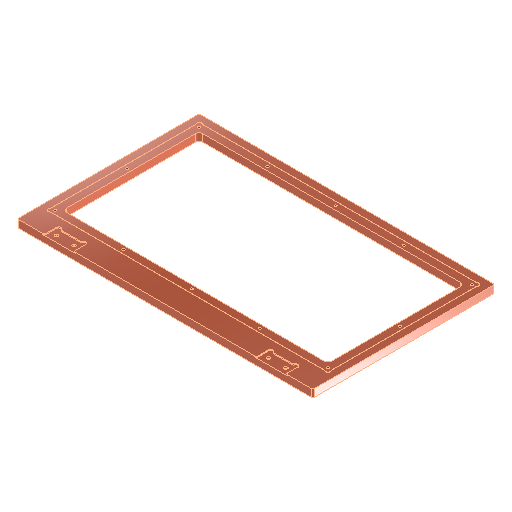
# Autodesk Inventor part: GRJ-04-105
Saved by Autodesk Inventor 2026.1 (Build 301233000, 233)
## iProperties
Company: Gree
Created: 2025-09-10
Part Number: GRJ-04-105
Material: Fenolite OR
Document SubType Name: Modeling
Designer: Willian Pinheiro
Density: 1.38 g/cm^3
Appearance: Suave - Laranja claro
Description: Suporte Estencil Principal
Project: GRJ-04
Mass: 415.457 g
Surface Area: 856.465 cm^2
Volume: 301.056 cm^3
Checked By: Antonio Lucas
Engr Approved By: Antonio Lucas
Mfg Approved By: Anderson Oliveira
Total: 1
Dimensões: 10 x 240 x 390 mm
Author: Willian Pinheiro
Title: Pasta Dissipador G
Revision Number: 00
Autodesk Inventor part; units mm, degrees
ref_plane "YZ Plane" through (0, 0, 0) normal (1, 0, 0) x (0, 1, 0)
ref_plane "XZ Plane" through (0, 0, 0) normal (0, 1, 0) x (-1, 0, 0)
ref_plane "XY Plane" through (0, 0, 0) normal (0, 0, 1) x (1, 0, 0)
sketch "Esboço1" plane through (0, 0, 0) normal (0, 0, 1) x (1, 0, 0)
  line L0 (-195, -120) -> (-195, 120)
  line L1 (-195, 120) -> (195, 120)
  line L2 (195, 120) -> (195, -120)
  line L3 (195, -120) -> (-195, -120)
  line L4 (0, 168.2) -> (0, -169.2) construction
  line L5 (-273, 0) -> (273, 0) construction
  line L6 (175, 100) -> (175, -80)
  line L7 (175, -80) -> (-175, -80)
  line L8 (-175, -80) -> (-175, 100)
  line L9 (-175, 100) -> (175, 100)
  line L10 (185, 110) -> (185, -90) construction
  line L11 (185, -90) -> (-185, -90) construction
  line L12 (-185, -90) -> (-185, 110) construction
  line L13 (-185, 110) -> (185, 110) construction
  line L14 (185.25, 110.25) -> (185.25, -90.25)
  line L15 (185.25, -90.25) -> (-185.25, -90.25)
  line L16 (-185.25, -90.25) -> (-185.25, 110.25)
  line L17 (-185.25, 110.25) -> (185.25, 110.25)
  circle A0 centre (183.25, 108.25) radius 3
  circle A1 centre (-183.25, 108.25) radius 3
  line L18 (175, 10) -> (-175, 10) construction
  circle A2 centre (183.25, -88.25) radius 3
  circle A3 centre (-183.25, -88.25) radius 3
  line L19 (180, 105) -> (180, -85) construction
  line L20 (180, -85) -> (-180, -85) construction
  line L21 (-180, -85) -> (-180, 105) construction
  line L22 (-180, 105) -> (180, 105) construction
  line L23 (159.5, -104) -> (159.5, -120)
  line L24 (159.5, -120) -> (120.5, -120)
  line L25 (120.5, -120) -> (120.5, -104)
  line L26 (120.5, -104) -> (159.5, -104)
  line L27 (140, -104) -> (140, -120) construction
  line L28 (159.5, -112) -> (120.5, -112) construction
  circle A4 centre (123.5, -104) radius 3
  line L29 (-159.5, -104) -> (-159.5, -120)
  line L30 (-159.5, -120) -> (-120.5, -120)
  line L31 (-120.5, -120) -> (-120.5, -104)
  line L32 (-120.5, -104) -> (-159.5, -104)
  line L33 (-140, -105) -> (-140, -121) construction
  line L34 (-159.5, -112) -> (-120.5, -112) construction
  circle A5 centre (-156.5, -104) radius 3
  circle A6 centre (-123.5, -104) radius 3
  circle A7 centre (156.5, -104) radius 3
  point P0 (0, 0)
  point P1 (0, -85)
  point P2 (-180, 10)
  point P3 (180, 10)
  point P4 (0, 105)
  point P5 (151.5, -112)
  point P6 (128.5, -112)
  point P7 (-151.5, -112)
  point P8 (-128.5, -112)
  point P9 (-181.0139, 110.25)
  point P10 (-185.25, 106.0139)
  point P11 (-185.25, -86.0139)
  point P12 (-181.0139, -90.25)
  point P13 (181.0139, -90.25)
  point P14 (185.25, -86.0139)
  point P15 (185.25, 106.0139)
  point P16 (181.0139, 110.25)
  point P17 (159.5, -120)
  point P18 (126.5, -104)
  point P19 (-153.5, -104)
  point P20 (-159.5, -120)
  point P21 (-126.5, -104)
  point P22 (-90, 105)
  point P23 (90, 105)
  point P24 (-90, -85)
  point P25 (90, -85)
  point P26 (106.5, -104)
  point P27 (153.5, -104)
  dimension "d112" = 10
  dimension "d113" = 0.25
  dimension "d114" = 6
  dimension "d115" = 2
  dimension "d116" = 2
  dimension "d117" = 5
  dimension "d123" = 16
  dimension "d124" = 8
  dimension "d125" = 39
  dimension "d126" = 280
  dimension "d127" = 240
  dimension "d128" = 390
  dimension "d129" = 20
  dimension "d130" = 200
  dimension "d131" = 350
  dimension "d132" = 10
  dimension "d133" = 0.25
  dimension "d134" = 5
  dimension "d163" = 90
  dimension "d164" = 90
  dimension "d165" = 23
  dimension "d166" = 370
  constraints: 62 end point, 12 midpoint, 7 centre point, 7 symmetric about line, 5 point on line, 4 coincident, 3 horizontal, 2 collinear, 1 parallel, 1 tangent, 28 other
  measures "d112" distance between parallel lines of L9 L13
  measures "d113" distance between parallel lines of L17 L13
  measures "d114" diameter of A0
  measures "d115" distance from line of A0.centre L17
  measures "d116" distance from line of A0.centre L14
  measures "d117" distance between parallel lines of L22 L9
  measures "d124" distance between parallel lines of L3 L34
  measures "d125" distance between parallel lines of L31 L29
  measures "d126" distance between parallel lines of L27 L33
  measures "d127" distance between parallel lines of L1 L3
  measures "d128" distance between parallel lines of L2 L0
  measures "d129" distance between parallel lines of L9 L1
  measures "d130" distance between parallel lines of L7 L1
  measures "d131" distance between parallel lines of L6 L8
  measures "d132" distance between parallel lines of L12 L8
  measures "d133" distance between parallel lines of L16 L12
  measures "d134" distance between parallel lines of L21 L8
  measures "d163" distance from line of point (-90, 105) L21
  measures "d164" distance of point (0, 105) point (-90, 105)
  measures "d165" distance of point (-128.5, -112) point (-151.5, -112)
  measures "d166" distance between parallel lines of L12 L10
extrude "Extrusão1" add sketch "Esboço1" against normal blind 10 contours L0 L1 L2 L3 L23 A7 L26 A4 L25 L31 A6 L32 A5 L29 | L29 A5 L32 A6 L31 L3 | A5 L32 | L32 A5 | L25 A4 L26 A7 L23 L3 | A6 L32 | L32 A6 | A4 L26 | L26 A4 | A7 L26 | L26 A7 | L6 L7 L8 L9 | L17 A0 L14 | L14 A0 L17 | L14 A2 L15 A3 L16 A1 L17 A0 | A2 L15 L14 | L14 L15 A2 | A1 L16 L17 | L17 L16 A1 | A3 L16 L15 | L15 L16 A3
extrude "Extrusion13" cut sketch "Esboço1" against normal blind 0.2 contours L6 L7 L8 L9 | L17 A0 L14 | L14 A0 L17 | L14 A2 L15 A3 L16 A1 L17 A0 | A2 L15 L14 | L14 L15 A2 | A1 L16 L17 | L17 L16 A1 | A3 L16 L15 | L15 L16 A3
extrude "Extrusion14" cut sketch "Esboço1" against normal blind 1.3 contours L29 A5 L32 A6 L31 L3 | A5 L32 | L32 A5 | L25 A4 L26 A7 L23 L3 | A6 L32 | L32 A6 | A4 L26 | L26 A4 | A7 L26 | L26 A7
extrude "Extrusion15" cut sketch "Esboço1" against normal through all contours L6 L7 L8 L9
hole "Hole4" at (-151.5, -112, 0) at (-128.5, -112, 0) at (128.5, -112, 0) at (151.5, -112, 0) direction (0, 0, -1) diameter 2.459 end through all thread size "M3x0.5" class "6H" standard "ISO Metric profile"
hole "Hole5" at (0, -85, 0) at (-180, -85, 0) at (-180, 10, 0) at (180, -85, 0) at (180, 10, 0) at (-180, 105, 0) at (0, 105, 0) at (180, 105, 0) at (90, -85, 0) at (90, 105, 0) at (-90, 105, 0) at (-90, -85, 0) direction (0, 0, -1) diameter 3.242 end through all thread size "M4x0.7" class "6H" standard "ISO Metric profile"
fillet "Fillet2" radius 2 20 edges at (-185.25, -86.0139, -0.1) (-181.0139, -90.25, -0.1) (-185.25, 106.0139, -0.1) (-181.0139, 110.25, -0.1) (181.0139, 110.25, -0.1) (185.25, 106.0139, -0.1) (181.0139, -90.25, -0.1) (185.25, -86.0139, -0.1) (-153.5, -104, -0.65) (-126.5, -104, -0.65) (195, -120, -5) (-195, -120, -5) (-195, 120, -5) (195, 120, -5) (153.5, -104, -0.65) (159.5, -120, -0.65) (120.5, -120, -0.65) (-159.5, -120, -0.65) (-120.5, -120, -0.65) (126.5, -104, -0.65)
fillet "Fillet2" radius 5 4 edges at (-175, 100, -5.1) (-175, -80, -5.1) (175, -80, -5.1) (175, 100, -5.1)
chamfer "Chamfer2" distance 1 angle 45 4 edges at (-151.5, -110.7705, -1.3) (-128.5, -110.7705, -1.3) (128.5, -110.7705, -1.3) (151.5, -110.7705, -1.3)
equation "\"d115\" = 0.333333 * d114"
equation "\"d116\" = d115"
